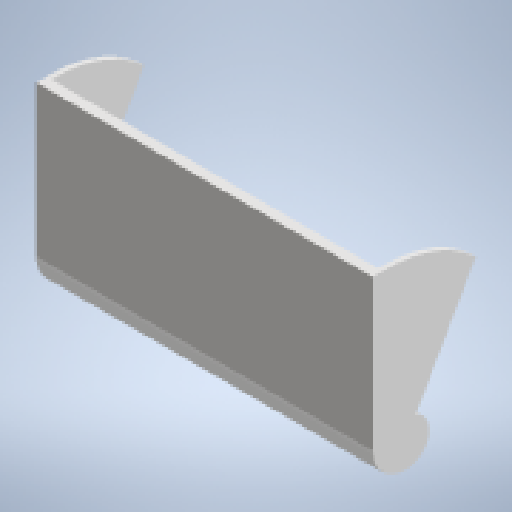
# Autodesk Inventor part: 후눈
Saved by Autodesk Inventor 2025 (Build 290162010, 162A)
## iProperties
Created: 2024-05-29
Part Number: 후눈
Material: 일반
Document SubType Name: Modeling
Designer: user
Density: 1 g/cm^3
Appearance: 기본값
Author: user
Autodesk Inventor part; units mm, degrees
ref_plane "YZ Plane" through (0, 0, 0) normal (1, 0, 0) x (0, 1, 0)
ref_plane "XZ Plane" through (0, 0, 0) normal (0, 1, 0) x (-1, 0, 0)
ref_plane "XY Plane" through (0, 0, 0) normal (0, 0, 1) x (1, 0, 0)
sketch "스케치1" plane through (0, 0, 0) normal (0, 0, 1) x (1, 0, 0)
  line L0 (70.1697, 650.1616) -> (730.1697, 650.1616)
  line L1 (730.1697, 650.1616) -> (730.1697, 290.1616)
  line L2 (730.1697, 290.1616) -> (70.1697, 290.1616)
  line L3 (70.1697, 290.1616) -> (70.1697, 650.1616)
  point P0 (0, 0)
  dimension "d0" = 660
  dimension "d1" = 360
  constraints: 8 end point, 2 parallel, 1 horizontal, 1 perpendicular
  measures "d0" distance of L1.end L2.end
  measures "d1" distance of L0.end L1.end
extrude "돌출1" add sketch "스케치1" along normal blind 20
sketch "스케치2" plane through (0, 0, 0) normal (0, 0, -1) x (-1, 0, 0)
  line L0 (-70.1697, 290.1616) -> (-730.1697, 290.1616) projected
  line L1 (-730.1697, 290.1616) -> (-720.1697, 290.1616)
  line L2 (-720.1697, 290.1616) -> (-720.1697, 380.1616)
  line L3 (-720.1697, 380.1616) -> (-730.1697, 380.1616)
  line L4 (-730.1697, 380.1616) -> (-730.1697, 290.1616)
  line L5 (-70.1697, 290.1616) -> (-80.1697, 290.1616)
  line L6 (-80.1697, 290.1616) -> (-80.1697, 380.1616)
  line L7 (-80.1697, 380.1616) -> (-70.1697, 380.1616)
  line L8 (-70.1697, 380.1616) -> (-70.1697, 290.1616)
  point P0 (0, 0)
  dimension "d4" = 10
  dimension "d5" = 90
  dimension "d6" = 10
  dimension "d7" = 90
  constraints: 16 end point, 4 parallel, 2 horizontal, 2 perpendicular
  measures "d4" distance of L3.end L2.end
  measures "d5" distance of L2.end L1.end
  measures "d6" distance of L6.end L7.end
  measures "d7" distance of L5.end L6.end
extrude "돌출2" add sketch "스케치2" along normal blind 90
fillet "모깎기1" radius 45 4 edges at (75.1697, 380.1616, -90) (75.1697, 290.1616, -90) (725.1697, 380.1616, -90) (725.1697, 290.1616, -90)
fillet "모깎기2" radius 65 1 edges at (400.1697, 290.1616, 20)
sketch "스케치3" plane through (70.1697, 650.1616, 0) normal (-1, 0, 0) x (0, 0, 1)
  arc A0 (0, 0) -> (-182.201, -66.335) centre (-7.9531, -261.5469) ccw
  line L0 (-182.201, -66.335) -> (-64.8769, -274.6279)
  arc A1 (-45, -270) -> (-45, -360) centre (-45, -315) ccw projected
  line L1 (0, -270) -> (0, 0)
  line L2 (-45, -270) -> (0, -270)
  arc A2 (-45, -270) -> (-64.8769, -274.6279) centre (-45, -315) ccw
  point P0 (0, -650.1616)
  constraints: 6 end point, 5 point on circle, 2 centre point, 2 tangent, 1 concentric, 1 perpendicular, 1 vertical
extrude "돌출3" add sketch "스케치3" against normal blind 10
sketch "스케치4" plane through (730.1697, 650.1616, 20) normal (1, 0, 0) x (0, 0, -1)
  arc A0 (65, -360) -> (84.8769, -274.6279) centre (65, -315) ccw projected
  arc A1 (202.201, -66.335) -> (20, 0) centre (27.9531, -261.5469) ccw projected
  line L0 (84.8769, -274.6279) -> (202.201, -66.335)
  arc A2 (202.201, -66.335) -> (20, 0) centre (27.9531, -261.5469) ccw
  line L1 (20, 0) -> (0, 0) projected
  line L2 (20, -270) -> (20, -341.9042) projected
  line L3 (20, 0) -> (20, -270)
  line L4 (20, -270) -> (65.7221, -270)
  arc A3 (84.8769, -274.6279) -> (65.7221, -270) centre (64.9878, -314.994) ccw
  point P0 (20, -650.1616)
  dimension "d14" = 45
  constraints: 6 end point, 4 point on circle, 2 centre point, 1 collinear, 1 concentric, 1 perpendicular
  measures "d14" radius of A3
extrude "돌출4" add sketch "스케치4" against normal blind 10
sketch "스케치5" plane through (730.1697, 355.1616, 20) normal (1, 0, 0) x (0, 0, -1)
  arc A0 (65, -65) -> (84.8769, 20.3721) centre (65, -20) ccw projected
  circle A1 centre (65, -20) radius 5
  point P0 (20, -355.1616)
  dimension "d17" = 10
  constraints: 1 centre point, 1 coincident
  measures "d17" diameter of A1
extrude "돌출5" add sketch "스케치5" along normal blind 10
sketch "스케치6" plane through (70.1697, 355.1616, 20) normal (-1, 0, 0) x (0, 0, 1)
  arc A0 (-84.8769, 20.3721) -> (-65, -65) centre (-65, -20) ccw projected
  circle A1 centre (-65, -20) radius 5
  point P0 (-20, -355.1616)
  dimension "d20" = 10
  constraints: 1 centre point, 1 coincident
  measures "d20" diameter of A1
extrude "돌출6" add sketch "스케치6" along normal blind 10
